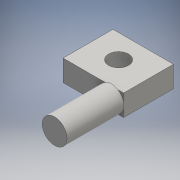
# Autodesk Inventor part: motor hombro
Saved by Autodesk Inventor 2016 (Build 200138000, 138)
## iProperties
Created: 2016-08-18
Part Number: motor hombro
Material: Generic
Document SubType Name: Modeling
Designer: Admin
Density: 1 g/cm^3
Appearance: Default
Author: Admin
Autodesk Inventor part; units mm, degrees
ref_plane "YZ Plane" through (0, 0, 0) normal (1, 0, 0) x (0, 1, 0)
ref_plane "XZ Plane" through (0, 0, 0) normal (0, 1, 0) x (-1, 0, 0)
ref_plane "XY Plane" through (0, 0, 0) normal (0, 0, 1) x (1, 0, 0)
sketch "Sketch1" plane through (0, 0, 0) normal (0, 1, 0) x (-1, 0, 0)
  circle A0 centre (0, 0) radius 17.5
  dimension "d0" = 35
  constraints: 1 centre point, 1 coincident
  measures "d0" diameter of A0
extrude "Extrusion1" add sketch "Sketch1" along normal blind 80
sketch "Sketch2" plane through (0, 80, 0) normal (0, 1, 0) x (1, 0, 0)
  line L0 (-68, -15) -> (17, -15)
  line L1 (17, -15) -> (17, 15)
  line L2 (17, 15) -> (-68, 15)
  line L3 (-68, 15) -> (-68, -15)
  point P0 (0, 0)
  dimension "d3" = 85
  dimension "d4" = 30
  constraints: 8 end point, 2 parallel, 1 horizontal, 1 perpendicular
  measures "d3" distance of L2.end L1.end
  measures "d4" distance of L1.end L0.end
extrude "Extrusion2" add sketch "Sketch2" along normal blind 70
sketch "Sketch3" plane through (-68, 80, 15) normal (0, 0, 1) x (1, 0, 0)
  circle A0 centre (41, 37) radius 14
  point P0 (68, -80)
  constraints: 1 centre point
extrude "Extrusion3" cut sketch "Sketch3" against normal through all
body "Solid1"
